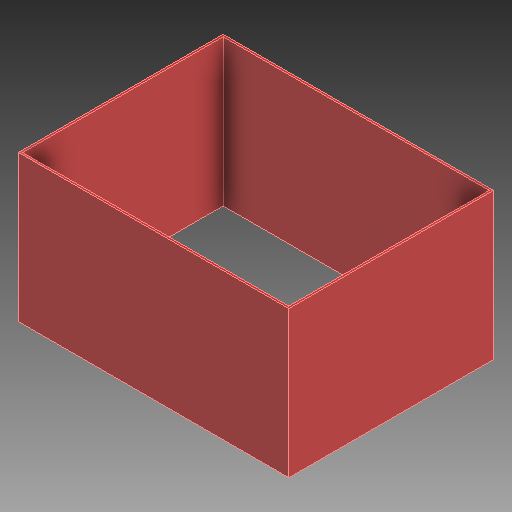
# Autodesk Inventor part: Back_ground
Saved by Autodesk Inventor 2023 (Build 270158000, 158)
## iProperties
Created: 2022-01-19
Part Number: Back_ground
Material: Типовые
Document SubType Name: Modeling
Designer: Администратор
Density: 1 g/cm^3
Appearance: Оранжево-красный
Author: Администратор
Autodesk Inventor part; units mm, degrees
ref_plane "YZ Plane" through (0, 0, 0) normal (1, 0, 0) x (0, 1, 0)
ref_plane "XZ Plane" through (0, 0, 0) normal (0, 1, 0) x (-1, 0, 0)
ref_plane "XY Plane" through (0, 0, 0) normal (0, 0, 1) x (1, 0, 0)
sketch "Эскиз1" plane through (0, 0, 0) normal (0, 1, 0) x (-1, 0, 0)
  line L0 (-1625.387, 869.9691) -> (844.613, 869.9691)
  line L1 (844.613, 869.9691) -> (844.613, -990.0309)
  line L2 (844.613, -990.0309) -> (-1625.387, -990.0309)
  line L3 (-1625.387, -990.0309) -> (-1625.387, 869.9691)
  line L4 (864.613, 889.9691) -> (-1645.387, 889.9691)
  line L5 (-1645.387, 889.9691) -> (-1645.387, -1010.0309)
  line L6 (-1645.387, -1010.0309) -> (864.613, -1010.0309)
  line L7 (864.613, -1010.0309) -> (864.613, 889.9691)
  point P0 (0, 0)
  dimension "d0" = 2470
  dimension "d1" = 1860
  dimension "d2" = 20
  constraints: 16 end point, 4 parallel, 2 perpendicular, 1 horizontal, 3 other
  measures "d0" distance of L0.start L0.end
  measures "d1" distance of L2.end L0.start
  measures "d2" distance between parallel lines of L0 L4
extrude "Выдавливание1" add sketch "Эскиз1" along normal blind 1359.75
